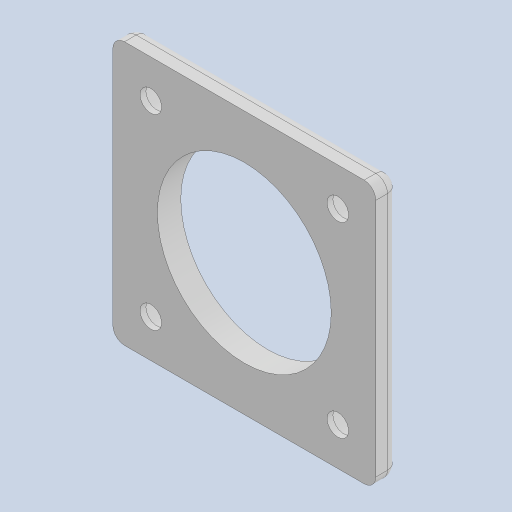
# Autodesk Inventor part: cage_inside_03
Saved by Autodesk Inventor 2024.4 (Build 284460000, 460)
## iProperties
Created: 2026-03-25
Part Number: cage_inside_03
Material: Generic
Document SubType Name: Modeling
Designer: tooles01
Density: 1 g/cm^3
Appearance: Default
Author: tooles01
Autodesk Inventor part; units mm, degrees
ref_plane "YZ Plane" through (0, 0, 0) normal (1, 0, 0) x (0, 1, 0)
ref_plane "XZ Plane" through (0, 0, 0) normal (0, 1, 0) x (-1, 0, 0)
ref_plane "XY Plane" through (0, 0, 0) normal (0, 0, 1) x (1, 0, 0)
sketch "Sketch1: base" plane through (0, 0, 0) normal (0, 0, 1) x (1, 0, 0)
  line L0 (-22.5, 22.5) -> (22.5, 22.5)
  line L1 (22.5, 22.5) -> (22.5, -22.5)
  line L2 (22.5, -22.5) -> (-22.5, -22.5)
  line L3 (-22.5, -22.5) -> (-22.5, 22.5)
  circle A0 centre (0, 0) radius 14.875
  line L4 (-16, 16) -> (16, 16) construction
  line L5 (16, 16) -> (16, -16) construction
  line L6 (16, -16) -> (-16, -16) construction
  line L7 (-16, -16) -> (-16, 16) construction
  circle A1 centre (16, 16) radius 1.8 construction
  circle A2 centre (16, 16) radius 3.25 construction
  point P0 (22.5, 0)
  point P1 (0, 22.5)
  point P2 (0, 16)
  point P3 (-16, 0)
  dimension "d0" = 29.75
  dimension "d1" = 45
  dimension "d4" = 32
  dimension "d19" = 6.5
  dimension "d20" = 3.6
  dimension "d21" = 6.5
  constraints: 16 end point, 8 perpendicular, 7 coincident, 4 midpoint, 3 centre point, 2 horizontal, 2 horizontal alignment, 2 vertical alignment
  measures "d0" diameter of A0
  measures "d1" distance of L0.start L0.end
  measures "d4" distance of L4.start L4.end
  measures "d19" distance between parallel lines of L1 L5
  measures "d20" diameter of A1
  measures "d21" diameter of A2
extrude "Ex1: base" add sketch "Sketch1: base" along normal blind 4
hole "Hole1: M3 screws" at (-16, 16, 0) at (16, 16, 0) at (-16, -16, 0) at (16, -16, 0) direction (0, 0, 1) diameter 3.7 end through all counterbore diameter 6.5 counterbore depth 3 clearance for "Socket Head Cap Screw" size "M3" standard "Ansi Metric M Profile"
fillet "Fillet1" radius 2 8 edges at (0, 22.5, 0) (22.5, 0, 0) (22.5, 22.5, 2) (-22.5, 0, 0) (0, -22.5, 0) (22.5, -22.5, 2) (-22.5, -22.5, 2) (-22.5, 22.5, 2)
sketch "Sketch2: text" plane through (0, 0, 0) normal (0, 0, -1) x (-1, 0, 0)
  line L0 (-9.5, 19) -> (-6, 19) construction
  line L1 (-6, 19) -> (-6, 15.5) construction
  line L2 (-6, 15.5) -> (-9.5, 15.5) construction
  line L3 (-9.5, 15.5) -> (-9.5, 19) construction
  line L4 (22.5, 22.5) -> (-22.5, 22.5) construction
  line L5 (-22.5, 22.5) -> (-22.5, -22.5) construction
  line L6 (22.5, -22.5) -> (22.5, 22.5) construction
  line L7 (-22.5, -22.5) -> (22.5, -22.5) construction
  circle A0 centre (-16, 16) radius 3.25 construction
  circle A1 centre (-16, 16) radius 1.8 construction
  line L8 (16, 16) -> (-16, 16) construction
  circle A2 centre (0, 0) radius 14.875 construction
  circle A3 centre (0, 0) radius 14.875 construction
  line L9 (-12.2062, 18.3737) -> (-10.7625, 18.3737)
  line L10 (-10.7625, 18.3737) -> (-10.0551, 16.0782)
  line L11 (-10.0551, 16.0782) -> (-9.3284, 18.3737)
  line L12 (-9.3284, 18.3737) -> (-7.9281, 18.3737)
  line L13 (-7.9281, 18.3737) -> (-9.468, 14.75)
  line L14 (-9.468, 14.75) -> (-10.7, 14.75)
  line L15 (-10.7, 14.75) -> (-12.2062, 18.3737)
  line L16 (-6.3111, 18.3063) -> (-7.6249, 18.5421)
  spline S0 degree 2 poles (-7.6249, 18.5421) (-7.4613, 19.1677) (-6.5325, 19.8366) (-5.6807, 19.8366) knots 0 0 0 1 2 2 2
  spline S1 degree 2 poles (-5.6807, 19.8366) (-4.699, 19.8366) (-3.828, 19.1051) (-3.828, 18.5565) knots 0 0 0 1 2 2 2
  spline S2 degree 2 poles (-3.828, 18.5565) (-3.828, 18.2293) (-4.1841, 17.7048) (-4.545, 17.5075) knots 0 0 0 1 2 2 2
  spline S3 degree 2 poles (-4.545, 17.5075) (-4.2514, 17.4353) (-4.0974, 17.339) knots 0 0 0 1 1 1
  spline S4 degree 2 poles (-4.0974, 17.339) (-3.8472, 17.185) (-3.5729, 16.6846) (-3.5729, 16.3381) knots 0 0 0 1 2 2 2
  spline S5 degree 2 poles (-3.5729, 16.3381) (-3.5729, 15.9001) (-4.0301, 15.0965) (-4.8867, 14.6634) (-5.5893, 14.6634) knots 0 0 0 1 2 3 3 3
  spline S6 degree 2 poles (-5.5893, 14.6634) (-6.2678, 14.6634) (-7.057, 14.9858) (-7.5671, 15.6018) (-7.7019, 16.0686) knots 0 0 0 1 2 3 3 3
  line L17 (-7.7019, 16.0686) -> (-6.3111, 16.2514)
  spline S7 degree 2 poles (-6.3111, 16.2514) (-6.2293, 15.8328) (-5.8876, 15.5103) (-5.623, 15.5103) knots 0 0 0 1 2 2 2
  spline S8 degree 2 poles (-5.623, 15.5103) (-5.3438, 15.5103) (-4.9733, 15.9194) (-4.9733, 16.2611) knots 0 0 0 1 2 2 2
  spline S9 degree 2 poles (-4.9733, 16.2611) (-4.9733, 16.6124) (-5.3294, 16.9925) (-5.6374, 16.9925) knots 0 0 0 1 2 2 2
  spline S10 degree 2 poles (-5.6374, 16.9925) (-5.801, 16.9925) (-6.0849, 16.9107) knots 0 0 0 1 1 1
  line L18 (-6.0849, 16.9107) -> (-6.0128, 17.9069)
  spline S11 degree 2 poles (-6.0128, 17.9069) (-5.8973, 17.8876) (-5.8347, 17.8876) knots 0 0 0 1 1 1
  spline S12 degree 2 poles (-5.8347, 17.8876) (-5.5604, 17.8876) (-5.1947, 18.2341) (-5.1947, 18.4747) knots 0 0 0 1 2 2 2
  spline S13 degree 2 poles (-5.1947, 18.4747) (-5.1947, 18.7009) (-5.469, 18.9752) (-5.7048, 18.9752) knots 0 0 0 1 2 2 2
  spline S14 degree 2 poles (-5.7048, 18.9752) (-5.9502, 18.9752) (-6.2582, 18.6769) (-6.3111, 18.3063) knots 0 0 0 1 2 2 2
  point P0 (-7.75, 19)
  point P1 (0, 22.5)
  dimension "d23" = 3.5
  dimension "d24" = 3.5
  dimension "d29" = 13
  constraints: 2 midpoint, 1 horizontal, 1 perpendicular, 2 other
  measures "d23" distance of L0.start L0.end
  measures "d24" distance between parallel lines of L4 L0
  measures "d29" distance between parallel lines of L5 L3
extrude "Ex3: text" cut sketch "Sketch2: text" against normal blind 1
body "Solid1"
